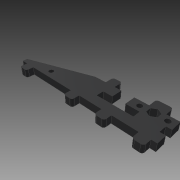
# Autodesk Inventor part: x_motor_wall_upper
Saved by Autodesk Inventor 2014 (Build 180170000, 170)
## iProperties
Created: 2013-12-01
Part Number: x_motor_wall_upper
Material: Generic
Document SubType Name: Modeling
Designer: buben
Density: 1 g/cm^3
Appearance: Anodized - Dark Gray
Author: buben
Subject: Laser Cutted
Autodesk Inventor part; units mm, degrees
ref_plane "YZ Plane" through (0, 0, 0) normal (1, 0, 0) x (0, 1, 0)
ref_plane "XZ Plane" through (0, 0, 0) normal (0, 1, 0) x (-1, 0, 0)
ref_plane "XY Plane" through (0, 0, 0) normal (0, 0, 1) x (1, 0, 0)
sketch "Sketch1" plane through (0, 0, 0) normal (0, 0, 1) x (1, 0, 0)
  line L0 (0, 4) -> (0, 0)
  line L1 (0, 0) -> (125, 0)
  line L2 (0, 4) -> (57, 23.5)
  line L3 (103, 14.5) -> (103, 8)
  line L4 (103, 8) -> (73, 8)
  line L5 (73, 8) -> (73, 14.5)
  line L6 (125, 14.5) -> (121, 14.5)
  line L7 (121, 14.5) -> (121, 8)
  line L8 (121, 8) -> (125, 8)
  line L9 (125, 0) -> (125, 8)
  line L10 (125, 14.5) -> (125, 23.5)
  line L11 (81, 23.5) -> (81, 14.5)
  line L12 (92, 14.5) -> (92, 23.5)
  line L13 (73, 14.5) -> (81, 14.5)
  line L14 (92, 14.5) -> (103, 14.5)
  line L15 (81, 14.5) -> (92, 14.5) construction
  circle A0 centre (86.5, 19.599) radius 7.5 construction
  circle A1 centre (86.5, 19.599) radius 4 construction
  line L16 (113.5, 21.9084) -> (113.5, 17.2896)
  line L17 (113.5, 17.2896) -> (109.5, 14.9802)
  line L18 (109.5, 14.9802) -> (105.5, 17.2896)
  line L19 (105.5, 17.2896) -> (105.5, 21.9084)
  line L20 (105.5, 21.9084) -> (109.5, 24.2178)
  line L21 (109.5, 24.2178) -> (113.5, 21.9084)
  circle A2 centre (109.5, 19.599) radius 2.5 construction
  line L22 (103.5, 23.5) -> (103.5, 29.5)
  line L23 (105.5, 31.5) -> (113.5, 31.5)
  line L24 (115.5, 29.5) -> (115.5, 23.5)
  arc A3 (105.5, 31.5) -> (103.5, 29.5) centre (105.5, 29.5) ccw
  arc A4 (115.5, 29.5) -> (113.5, 31.5) centre (113.5, 29.5) ccw
  line L25 (125, 23.5) -> (115.5, 23.5)
  line L26 (103.5, 23.5) -> (92, 23.5)
  circle A5 centre (99.5, 19) radius 4.5 construction
  circle A6 centre (119.5, 19) radius 4.5 construction
  circle A7 centre (99.5, 19) radius 2.25
  circle A8 centre (119.5, 19) radius 2.25
  line L27 (67, 23.5) -> (67, 29.5)
  line L28 (69, 31.5) -> (73, 31.5)
  line L29 (75, 29.5) -> (75, 23.5)
  arc A9 (69, 31.5) -> (67, 29.5) centre (69, 29.5) ccw
  arc A10 (75, 29.5) -> (73, 31.5) centre (73, 29.5) ccw
  line L30 (81, 23.5) -> (75, 23.5)
  line L31 (67, 23.5) -> (57, 23.5)
  point P0 (81, 14.5)
  point P1 (92, 14.5)
  point P2 (86.5, 14.5)
  point P3 (125, 19)
  point P4 (109.5, 31.5)
  dimension "d0" = 8
  dimension "d2" = 6.5
  dimension "d3" = 4
  dimension "d4" = 15
  dimension "d5" = 8
  dimension "d6" = 9
  dimension "d7" = 11
  dimension "d8" = 11
  dimension "d9" = 8
  dimension "d10" = 5
  dimension "d11" = 2
  dimension "d12" = 12
  dimension "d13" = 9
  dimension "d14" = 9
  dimension "d15" = 10
  dimension "d16" = 10
  dimension "d17" = 4.5
  dimension "d18" = 4.5
  dimension "d19" = 13
  dimension "d20" = 5.5
  dimension "d21" = 18
  dimension "d22" = 2
  dimension "d23" = 8
  dimension "d24" = 6
  dimension "d25" = 10
  dimension "d27" = 30
  dimension "d28" = 4
  dimension "d30" = 8
  dimension "d31" = 125
  constraints: 64 end point, 23 perpendicular, 11 centre point, 10 collinear, 10 point on circle, 9 parallel, 8 tangent, 4 coincident, 3 horizontal alignment, 3 midpoint, 2 equal radius, 2 horizontal, 2 point on line, 2 vertical alignment, 1 vertical, 13 other
  measures "d0" distance between parallel lines of L1 L4
  measures "d2" distance of L3.start L3.end
  measures "d3" distance of L7.end L8.end
  measures "d4" diameter of A0
  measures "d5" diameter of A1
  measures "d6" distance of L12.start L12.end
  measures "d7" distance of A0.end A0.start
  measures "d8" distance between parallel lines of L12 L11
  measures "d9" distance between parallel lines of L16 L19
  measures "d10" diameter of A2
  measures "d11" radius of A3
  measures "d12" distance between parallel lines of L24 L22
  measures "d13" diameter of A5
  measures "d14" diameter of A6
  measures "d15" horizontal distance of point (109.5, 19.599) A6.centre
  measures "d16" horizontal distance of point (109.5, 19.599) A5.centre
  measures "d17" diameter of A7
  measures "d18" diameter of A8
  measures "d19" horizontal distance of A5.centre A0.centre
  measures "d20" distance from line of L10 A6.centre
  measures "d21" distance between parallel lines of L7 L3
  measures "d22" radius of A9
  measures "d23" distance between parallel lines of L29 L27
  measures "d24" distance of L11.start L29.end
  measures "d25" distance of L27.start L2.end
  measures "d27" distance of L3.end L4.end
  measures "d28" distance of L0.start L0.end
  measures "d30" distance between parallel lines of L31 L28
  measures "d31" distance of L0.end L1.end
extrude "Extrusion1" add sketch "Sketch1" along normal blind 6.5
sketch "Sketch2" plane through (0, 0, 6.5) normal (0, 0, 1) x (1, 0, 0)
  line L0 (0, 4) -> (0, 0) projected
  line L1 (0, 0) -> (125, 0) projected
  line L2 (6, 0) -> (14, 0)
  line L3 (14, 0) -> (14, -4.5)
  line L4 (12, -6.5) -> (8, -6.5)
  line L5 (6, -4.5) -> (6, 0)
  line L6 (57, 0) -> (65, 0)
  line L7 (65, 0) -> (65, -4.5)
  line L8 (63, -6.5) -> (59, -6.5)
  line L9 (57, -4.5) -> (57, 0)
  line L10 (85, 0) -> (93, 0)
  line L11 (93, 0) -> (93, -4.5)
  line L12 (91, -6.5) -> (87, -6.5)
  line L13 (85, -4.5) -> (85, 0)
  line L14 (113, 0) -> (121, 0)
  line L15 (121, 0) -> (121, -4.5)
  line L16 (119, -6.5) -> (115, -6.5)
  line L17 (113, -4.5) -> (113, 0)
  arc A0 (6, -4.5) -> (8, -6.5) centre (8, -4.5) ccw
  arc A1 (12, -6.5) -> (14, -4.5) centre (12, -4.5) ccw
  arc A2 (57, -4.5) -> (59, -6.5) centre (59, -4.5) ccw
  arc A3 (63, -6.5) -> (65, -4.5) centre (63, -4.5) ccw
  arc A4 (85, -4.5) -> (87, -6.5) centre (87, -4.5) ccw
  arc A5 (91, -6.5) -> (93, -4.5) centre (91, -4.5) ccw
  arc A6 (113, -4.5) -> (115, -6.5) centre (115, -4.5) ccw
  arc A7 (119, -6.5) -> (121, -4.5) centre (119, -4.5) ccw
  dimension "d34" = 2
  dimension "d35" = 8
  dimension "d36" = 8
  dimension "d37" = 8
  dimension "d38" = 8
  dimension "d39" = 6.5
  dimension "d40" = 6
  dimension "d41" = 43
  dimension "d42" = 20
  dimension "d43" = 20
  constraints: 32 end point, 16 point on circle, 16 tangent, 8 centre point, 8 parallel, 7 equal radius, 4 horizontal, 4 perpendicular, 4 point on line, 3 collinear
  measures "d34" radius of A0
  measures "d35" distance between parallel lines of L3 L5
  measures "d36" distance between parallel lines of L7 L9
  measures "d37" distance between parallel lines of L11 L13
  measures "d38" distance between parallel lines of L15 L17
  measures "d39" distance between parallel lines of L1 L4
  measures "d40" distance between parallel lines of L0 L5
  measures "d41" distance between parallel lines of L9 L3
  measures "d42" distance between parallel lines of L13 L7
  measures "d43" distance between parallel lines of L17 L11
extrude "Extrusion2" add sketch "Sketch2" against normal blind 6.5
sketch "Sketch3" plane through (0, 0, 6.5) normal (0, 0, 1) x (1, 0, 0)
  line L0 (0, 4) -> (0, 0) projected
  line L1 (14, 0) -> (57, 0) projected
  circle A0 centre (28.2, 6) radius 2.25
  circle A1 centre (28.2, 6) radius 4.5 construction
  dimension "d46" = 4.5
  dimension "d47" = 6
  dimension "d48" = 28.2
  dimension "d51" = 9
  constraints: 2 centre point, 1 coincident
  measures "d46" diameter of A0
  measures "d47" distance from line of L1 A0.centre
  measures "d48" distance from line of L0 A0.centre
  measures "d51" diameter of A1
extrude "Extrusion3" cut sketch "Sketch3" against normal through all
body "Solid1"
